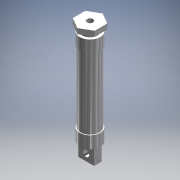
# Autodesk Inventor part: 50mm Cylinder
Saved by Autodesk Inventor 2019.4 (Build 234330000, 330)
## iProperties
Created: 2020-01-29
Part Number: 50mm Cylinder
Material: Aluminum 6061
Document SubType Name: Modeling
Designer: admin
Density: 2.7 g/cm^3
Appearance: Aluminum - Flat
Mass: 195.849 g
Surface Area: 159.624 cm^2
Volume: 72.5368 cm^3
Author: admin
Autodesk Inventor part; units mm, degrees
ref_plane "YZ Plane" through (0, 0, 0) normal (1, 0, 0) x (0, 1, 0)
ref_plane "XZ Plane" through (0, 0, 0) normal (0, 1, 0) x (-1, 0, 0)
ref_plane "XY Plane" through (0, 0, 0) normal (0, 0, 1) x (1, 0, 0)
sketch "Sketch1" plane through (0, 0, 0) normal (0, 1, 0) x (-1, 0, 0)
  circle A0 centre (0, 0) radius 13.5
  dimension "d0" = 27
  constraints: 1 centre point, 1 coincident
  measures "d0" diameter of A0
extrude "Extrusion1" add sketch "Sketch1" along normal blind 16
sketch "Sketch2" plane through (0, 16, 0) normal (0, 1, 0) x (1, 0, 0)
  circle A0 centre (0, 0) radius 12.5
  dimension "d3" = 25
  constraints: 1 centre point, 1 coincident
  measures "d3" diameter of A0
extrude "Extrusion2" add sketch "Sketch2" along normal blind 94
sketch "Sketch3" plane through (0, 110, 0) normal (0, 1, 0) x (1, 0, 0)
  circle A0 centre (0, 0) radius 13.5
  dimension "d6" = 27
  constraints: 1 centre point, 1 coincident
  measures "d6" diameter of A0
extrude "Extrusion3" add sketch "Sketch3" along normal blind 16
sketch "Sketch5" plane through (0, 126, 0) normal (0, 1, 0) x (1, 0, 0)
  circle A0 centre (0, 0) radius 10
  dimension "d12" = 20
  constraints: 1 centre point, 1 coincident
  measures "d12" diameter of A0
extrude "Extrusion5" add sketch "Sketch5" along normal blind 5
sketch "Sketch4" plane through (0, 131, 0) normal (0, 1, 0) x (1, 0, 0)
  line L0 (0, 16.7432) -> (14.5, 8.3716)
  line L1 (14.5, 8.3716) -> (14.5, -8.3716)
  line L2 (14.5, -8.3716) -> (0, -16.7432)
  line L3 (0, -16.7432) -> (-14.5, -8.3716)
  line L4 (-14.5, -8.3716) -> (-14.5, 8.3716)
  line L5 (-14.5, 8.3716) -> (0, 16.7432)
  point P0 (0, 0)
  point P1 (0, 0)
  dimension "d9" = 29
  constraints: 12 end point, 1 coincident, 1 vertical, 13 other
  measures "d9" distance between parallel lines of L1 L4
extrude "Extrusion4" add sketch "Sketch4" along normal blind 7
sketch "Sketch6" plane through (0, 138, 0) normal (0, 1, 0) x (1, 0, 0)
  circle A0 centre (0, 0) radius 4
  dimension "d15" = 8
  constraints: 1 centre point, 1 coincident
  measures "d15" diameter of A0
extrude "Extrusion6" [suppressed]
sketch "Sketch7" plane through (0, 146, 0) normal (0, 1, 0) x (1, 0, 0)
  circle A0 centre (0, 0) radius 4.4
  dimension "d18" = 8.8
  constraints: 1 centre point, 1 coincident
  measures "d18" diameter of A0
extrude "Extrusion7" [suppressed]
sketch "Sketch8" plane through (0, 153, 0) normal (0, 1, 0) x (1, 0, 0)
  line L0 (0, 9.2376) -> (8, 4.6188)
  line L1 (8, 4.6188) -> (8, -4.6188)
  line L2 (8, -4.6188) -> (0, -9.2376)
  line L3 (0, -9.2376) -> (-8, -4.6188)
  line L4 (-8, -4.6188) -> (-8, 4.6188)
  line L5 (-8, 4.6188) -> (0, 9.2376)
  point P0 (0, 0)
  point P1 (0, 0)
  dimension "d21" = 16
  constraints: 12 end point, 1 coincident, 1 vertical, 13 other
  measures "d21" distance between parallel lines of L1 L4
extrude "Extrusion8" [suppressed]
sketch "Sketch9" plane through (0, 159, 0) normal (0, 1, 0) x (1, 0, 0)
  circle A0 centre (0, 0) radius 4.4
  dimension "d24" = 8.8
  constraints: 1 centre point, 1 coincident
  measures "d24" diameter of A0
extrude "Extrusion9" [suppressed]
thread "Thread1" size "M9x1.25" class "6g" standard "ANSI Metric M Profile" full length
sketch "Sketch10" plane through (0, 0, 0) normal (0, -1, 0) x (1, 0, 0)
  line L0 (-10.5, -5.0125) -> (10.5, -5.0125)
  line L1 (10.5, -5.0125) -> (10.5, 5.0125)
  line L2 (10.5, 5.0125) -> (-10.5, 5.0125)
  line L3 (-10.5, 5.0125) -> (-10.5, -5.0125)
  line L4 (-10.5, -5.0125) -> (10.5, 5.0125) construction
  line L5 (10.5, -5.0125) -> (-10.5, 5.0125) construction
  point P0 (0, 0)
  dimension "d29" = 21
  constraints: 12 end point, 2 midpoint, 2 parallel, 1 horizontal, 1 perpendicular
  measures "d29" distance of L0.start L0.end
extrude "Extrusion10" add sketch "Sketch10" along normal blind 21
sketch "Sketch11" plane through (-10.5, 0, 5.0125) normal (0, 0, 1) x (1, 0, 0)
  circle A0 centre (10.5, -12) radius 4
  line L0 (21, -21) -> (0, -21) projected
  line L1 (-3, 0) -> (24, 0) projected
  line L2 (10.5, -12) -> (10.5, -21) construction
  point P0 (10.5, 0)
  dimension "d32" = 8
  dimension "d34" = 12
  constraints: 2 end point, 1 centre point, 1 midpoint, 1 vertical
  measures "d32" diameter of A0
  measures "d34" distance from line of L1 L2.start
extrude "Extrusion11" cut sketch "Sketch11" against normal through all
sketch "Sketch12" plane through (0, 138, 0) normal (0, 1, 0) x (1, 0, 0)
  circle A0 centre (0, 0) radius 13.5 projected
  constraints: 1 coincident
hole "Hole1" at (0, 138, 0) direction (0, -1, 0) diameter 8 depth 50
body "Solid1"
